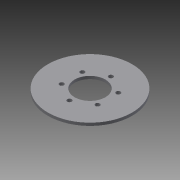
# Autodesk Inventor part: Strap Shield
Saved by Autodesk Inventor 2013 (Build 170138000, 138)
## iProperties
Created: 2014-02-03
Part Number: Strap Shield
Material: Generic
Document SubType Name: Modeling
Designer: sethbattis
Density: 1 g/cm^3
Author: sethbattis
Autodesk Inventor part; units mm, degrees
ref_plane "YZ Plane" through (0, 0, 0) normal (1, 0, 0) x (0, 1, 0)
ref_plane "XZ Plane" through (0, 0, 0) normal (0, 1, 0) x (-1, 0, 0)
ref_plane "XY Plane" through (0, 0, 0) normal (0, 0, 1) x (1, 0, 0)
sketch "Sketch1" plane through (0, 0, 0) normal (0, 1, 0) x (-1, 0, 0)
  circle A0 centre (0, 0) radius 17.4625
  line L0 (115.2587, 0) -> (-115.7035, 0) construction
  line L1 (-0.2224, 95.1184) -> (82.2641, -47.7524) construction
  line L2 (82.2641, -47.7524) -> (-82.7089, -47.7524) construction
  line L3 (-82.7089, -47.7524) -> (-0.2224, 95.1184) construction
  line L4 (0, 0) -> (-41.4657, 23.683) construction
  line L5 (0, 0) -> (37.9918, 28.9294) construction
  line L6 (0, 0) -> (0, -47.7524) construction
  circle A1 centre (0, 0) radius 47.7524
  line L7 (-0.1924, 23.525) -> (-0.1924, -23.525) construction
  circle A2 centre (-0.1924, 23.525) radius 2.5
  circle A3 centre (-0.1924, -23.525) radius 2.5
  line L8 (0, 0) -> (-18.1393, 10.4727) construction
  circle A4 centre (0, 0) radius 23.5258 construction
  circle A5 centre (-20.3739, 11.7629) radius 2.5
  line L9 (-0.1924, 21.025) -> (5.7447, 21.025) construction
  line L10 (-0.1924, -21.025) -> (5.7447, -21.025) construction
  line L11 (0, 0) -> (-31.1741, -17.9984) construction
  circle A6 centre (-20.3739, -11.7629) radius 2.5
  line L12 (0, 0) -> (30.9754, -17.8837) construction
  line L13 (0, 0) -> (26.3932, 15.2381) construction
  circle A7 centre (20.3739, 11.7629) radius 2.5
  circle A8 centre (20.3739, -11.7629) radius 2.5
  dimension "d16" = 5
  dimension "d17" = 5
  dimension "d0" = 34.925
  dimension "d5" = 164.973
  dimension "d18" = 60
  dimension "d19" = 5
  dimension "d20" = 42.05
  dimension "d21" = 5
  dimension "d22" = 60
  dimension "d23" = 5
  dimension "d24" = 5
  dimension "d25" = 60
  dimension "d26" = 60
  constraints: 26 end point, 11 point on line, 6 centre point, 6 point on circle, 4 coincident, 4 equal length, 3 perpendicular, 2 horizontal, 2 parallel, 2 vertical alignment, 1 midpoint, 1 symmetric about line, 8 other
  measures "d0" diameter of A0
  measures "d5" distance of L2.end L1.start
  measures "d18" angle of L8 L7
  measures "d19" diameter of A5
  measures "d20" distance between parallel lines of L9 L10
  measures "d21" diameter of A6
  measures "d22" angle of L7 L11
  measures "d23" diameter of A7
  measures "d24" diameter of A8
  measures "d25" angle of L12 L7
  measures "d26" angle of L13 L12
extrude "Extrusion2" add sketch "Sketch1" along normal blind 3.175
body "Solid2"
